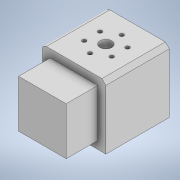
# Autodesk Inventor part: BasicCube
Saved by Autodesk Inventor 2022 (Build 260153000, 153)
## iProperties
Created: 2021-09-22
Part Number: BasicCube
Material: Generic
Document SubType Name: Modeling
Designer: merky
Density: 1 g/cm^3
Appearance: Default
Author: merky
Autodesk Inventor part; units mm, degrees
ref_plane "YZ Plane" through (0, 0, 0) normal (1, 0, 0) x (0, 1, 0)
ref_plane "XZ Plane" through (0, 0, 0) normal (0, 1, 0) x (-1, 0, 0)
ref_plane "XY Plane" through (0, 0, 0) normal (0, 0, 1) x (1, 0, 0)
sketch "Sketch1" plane through (0, 0, 0) normal (0, 1, 0) x (-1, 0, 0)
  line L0 (0, 0) -> (101.6, 0)
  line L1 (101.6, 0) -> (101.6, -101.6)
  line L2 (101.6, -101.6) -> (0, -101.6)
  line L3 (0, -101.6) -> (0, 0)
  dimension "d0" = 101.6
  dimension "d1" = 101.6
  constraints: 8 end point, 2 parallel, 1 horizontal, 1 perpendicular
  measures "d0" distance of L1.end L2.end
  measures "d1" distance of L0.end L1.end
extrude "Extrusion1" add sketch "Sketch1" along normal blind 101.6
sketch "Sketch2" plane through (0, 101.6, 0) normal (0, 1, 0) x (1, 0, 0)
  circle A0 centre (-50.8, 50.8) radius 9.4395
  point P0 (0, 0)
  point P1 (-50.8, 25.4)
  point P2 (-28.803, 38.1)
  point P3 (-28.803, 63.5)
  point P4 (-50.8, 76.2)
  point P5 (-72.797, 63.5)
  point P6 (-72.797, 38.1)
  dimension "d6" = 360
  constraints: 1 centre point, 1 coincident, 7 other
extrude "Extrusion2" cut sketch "Sketch2" against normal through all
hole "Hole1" at (-50.8, 101.6, -50.8) at (-50.8, 101.6, -25.4) at (-28.803, 101.6, -38.1) at (-28.803, 101.6, -63.5) at (-50.8, 101.6, -76.2) at (-72.797, 101.6, -63.5) at (-72.797, 101.6, -38.1) direction (0, -1, 0) diameter 6.35 end through all
fillet "Fillet1" radius 6.35 1 edges at (-101.6, 101.6, -50.8)
chamfer "Chamfer1" distance 6.35 angle 45 1 edges at (0, 101.6, -50.8)
sketch "Sketch3" plane through (-101.6, 0, 0) normal (0, 0, 1) x (1, 0, 0)
  line L0 (12.7, 88.9) -> (88.9, 88.9)
  line L1 (88.9, 88.9) -> (88.9, 12.7)
  line L2 (88.9, 12.7) -> (12.7, 12.7)
  line L3 (12.7, 12.7) -> (12.7, 88.9)
  line L4 (12.7, 88.9) -> (88.9, 12.7) construction
  line L5 (88.9, 88.9) -> (12.7, 12.7) construction
  point P0 (101.6, 0)
  point P1 (50.8, 50.8)
  dimension "d21" = 76.2
  dimension "d22" = 76.2
  constraints: 12 end point, 2 midpoint, 2 parallel, 1 horizontal, 1 perpendicular
  measures "d21" distance of L1.end L2.end
  measures "d22" distance of L0.end L1.end
extrude "Extrusion3" add sketch "Sketch3" along normal blind 50.8
body "Solid1"
